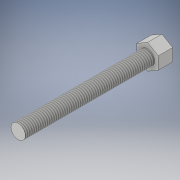
# Autodesk Inventor part: 4 in bolt
Saved by Autodesk Inventor 2017 (Build 210142000, 142)
## iProperties
Created: 2017-05-26
Part Number: 4 in bolt
Material: Generic
Document SubType Name: Modeling
Designer: cas7
Density: 1 g/cm^3
Appearance: Default
Author: cas7
Autodesk Inventor part; units mm, degrees
ref_plane "YZ Plane" through (0, 0, 0) normal (1, 0, 0) x (0, 1, 0)
ref_plane "XZ Plane" through (0, 0, 0) normal (0, 1, 0) x (-1, 0, 0)
ref_plane "XY Plane" through (0, 0, 0) normal (0, 0, 1) x (1, 0, 0)
sketch "Sketch1" plane through (0, 0, 0) normal (0, 0, 1) x (1, 0, 0)
  circle A0 centre (0, 0) radius 6.35
  line L0 (0, 10.9985) -> (9.525, 5.4993)
  line L1 (9.525, 5.4993) -> (9.525, -5.4993)
  line L2 (9.525, -5.4993) -> (0, -10.9985)
  line L3 (0, -10.9985) -> (-9.525, -5.4993)
  line L4 (-9.525, -5.4993) -> (-9.525, 5.4993)
  line L5 (-9.525, 5.4993) -> (0, 10.9985)
  dimension "d1" = 19.05
  constraints: 12 end point, 2 coincident, 1 centre point, 13 other
  measures "d1" distance between parallel lines of L3 L0
extrude "Extrusion1" add sketch "Sketch1" against normal blind 12.7 contours A0 | L0 L1 L2 L3 L4 L5
sketch "Sketch2" plane through (0, 0, 0) normal (0, 0, 1) x (1, 0, 0)
  circle A0 centre (0, 0) radius 6.35
  dimension "d4" = 12.7
  constraints: 1 centre point, 1 coincident
  measures "d4" diameter of A0
extrude "Extrusion2" add sketch "Sketch2" along normal blind 114.3
thread "Thread1" size "1/2-13 UNC" class "2A" standard "ANSI Unified Screw Threads" full length
body "Solid1"
